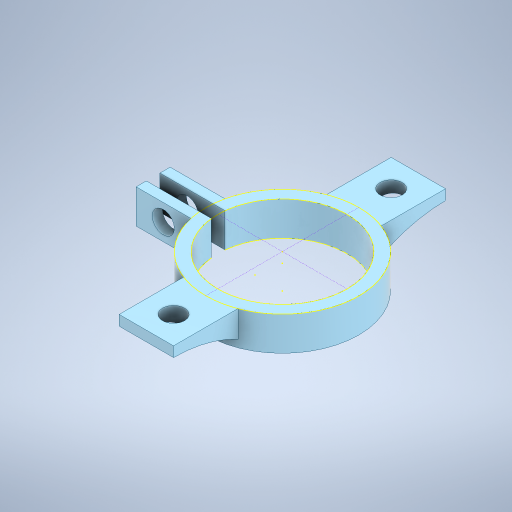
# Autodesk Inventor part: motor holder
Saved by Autodesk Inventor 2023 (Build 270158000, 158)
## iProperties
Created: 2023-04-19
Part Number: motor holder
Material: ABS Plastic
Document SubType Name: Modeling
Designer: deepa
Density: 1.06 g/cm^3
Appearance: Smooth - White
Author: deepa
Autodesk Inventor part; units mm, degrees
ref_plane "YZ Plane" through (0, 0, 0) normal (1, 0, 0) x (0, 1, 0)
ref_plane "XZ Plane" through (0, 0, 0) normal (0, 1, 0) x (-1, 0, 0)
ref_plane "XY Plane" through (0, 0, 0) normal (0, 0, 1) x (1, 0, 0)
sketch "Sketch1" plane through (0, 0, 0) normal (0, 1, 0) x (-1, 0, 0)
  circle A0 centre (0, 0) radius 22.5
  circle A1 centre (0, 0) radius 19
  dimension "d0" = 45
  dimension "d1" = 38
  constraints: 2 centre point, 1 coincident
  measures "d0" diameter of A0
  measures "d1" diameter of A1
extrude "Extrusion1" add sketch "Sketch1" along normal blind 10
sketch "Sketch2" plane through (0, 10, 0) normal (0, 1, 0) x (1, 0, 0)
  circle A0 centre (0, 0) radius 22.5 projected
  line L0 (0, -22.5) -> (0, 22.5) construction
  circle A1 centre (0, 0) radius 19 projected
  line L1 (-19, 0) -> (19, 0) construction
  constraints: 4 end point, 4 point on circle, 1 horizontal, 1 vertical
sketch "Sketch3" plane through (0, 10, 0) normal (0, 1, 0) x (1, 0, 0)
  line L0 (-8, -20) -> (8, -20)
  line L1 (8, -20) -> (8, -40)
  line L2 (8, -40) -> (-8, -40)
  line L3 (-8, -40) -> (-8, -20)
  point P0 (0, 0)
  dimension "d4" = 16
  dimension "d5" = 20
  dimension "d6" = 20
  dimension "d7" = 8
  constraints: 8 end point, 2 parallel, 1 horizontal, 1 perpendicular
  measures "d4" distance of L1.end L2.end
  measures "d5" distance from line of L0 point (0, 0)
  measures "d6" distance of L2.end L0.start
  measures "d7" distance from line of L3 point (0, 0)
extrude "Extrusion2" add sketch "Sketch3" against normal blind 3
pattern_circular "Circular Pattern1" count 2 over 360 about axis through (0, 0, 0) along (0, 1, 0) of "Extrusion2"
sketch "Sketch4" plane through (0, 10, 0) normal (0, 1, 0) x (1, 0, 0)
  point P0 (0, 0)
sketch "Sketch6" plane through (0, 10, 0) normal (0, 1, 0) x (1, 0, 0)
  line L0 (-20, 5) -> (-38, 5)
  line L1 (-38, 5) -> (-38, 2)
  line L2 (-38, 2) -> (-20, 2)
  line L3 (-20, 2) -> (-20, 5)
  point P0 (0, 0)
  dimension "d14" = 18
  dimension "d15" = 3
  dimension "d16" = 20
  dimension "d17" = 2
  constraints: 8 end point, 2 parallel, 1 horizontal, 1 perpendicular
  measures "d14" distance of L2.end L1.end
  measures "d15" distance of L1.end L0.end
  measures "d16" distance from line of L3 point (0, 0)
  measures "d17" distance from line of L2 point (0, 0)
extrude "Extrusion3" add sketch "Sketch6" against normal blind 10
pattern_linear "Rectangular Pattern1" count 2 spacing 7 along (0, 0, 1) of "Extrusion3"
sketch "Sketch7" plane through (-38, 10, 2) normal (-1, 0, 0) x (0, 0, 1)
  line L0 (0, 0) -> (0, -10) projected
  line L1 (-4, 0) -> (-4, -10) projected
  line L2 (0, -10) -> (-4, -10)
  line L3 (-4, -10) -> (-4, 0)
  line L4 (-4, 0) -> (0, 0)
  line L5 (0, 0) -> (0, -10)
  point P0 (-2, -10)
  constraints: 8 end point, 2 parallel, 1 horizontal, 1 perpendicular
extrude "Extrusion4" cut sketch "Sketch7" against normal blind 20
sketch "Sketch9" plane through (0, 7, 0) normal (0, -1, 0) x (1, 0, 0)
  point P0 (0, 0)
sketch "Sketch10" plane through (0, 7, 0) normal (0, -1, 0) x (1, 0, 0)
  point P0 (0, 0)
sketch "Sketch11" plane through (8, 10, -40) normal (0, 0, -1) x (-1, 0, 0)
  point P0 (8, -10)
sketch "Sketch13" plane through (-8, 10, -40) normal (-1, 0, 0) x (0, 0, 1)
  point P0 (40, -10)
sketch "Sketch14" plane through (-38, 10, 5) normal (0, 0, 1) x (1, 0, 0)
  circle A0 centre (8, -5) radius 3.25
  line L0 (0, 0) -> (0, -10) projected
  line L1 (16.0626, -10) -> (0, -10) projected
  point P0 (38, -10)
  dimension "d27" = 6.5
  dimension "d28" = 8
  dimension "d29" = 5
  constraints: 1 centre point
  measures "d27" diameter of A0
  measures "d28" distance from line of L0 A0.centre
  measures "d29" distance from line of L1 A0.centre
extrude "Extrusion5" cut sketch "Sketch14" against normal blind 20
sketch "Sketch17" plane through (0, 0, 0) normal (0, -1, 0) x (1, 0, 0)
  arc A0 (-21.9374, -5) -> (-8, -21.0297) centre (0, 0) ccw projected
  line L0 (-8, -21.0297) -> (-8, -17.2337) construction
  arc A1 (-18.8944, -2) -> (-18.8944, 2) centre (0, 0) ccw projected
  constraints: 2 end point, 1 point on circle, 1 vertical
sketch "Sketch21" plane through (-8, 10, -40) normal (-1, 0, 0) x (0, 0, 1)
  line L0 (0, -43) -> (18, -10) construction
  line L1 (62.5, -10) -> (17.5, -10) projected
  line L2 (18.9703, -3) -> (0, -3) projected
  line L3 (0, 0) -> (0, -3) projected
  circle A0 centre (0, -43) radius 40
  line L4 (18.9703, -3) -> (18.9703, -10)
  point P0 (40, -10)
  point P1 (45, -10)
  point P2 (35, -10)
  point P3 (18.9703, -7.7845)
  dimension "d33" = 40
  dimension "d34" = 0
  dimension "d35" = 18
  constraints: 4 end point, 2 point on line, 1 centre point, 1 coincident, 1 perpendicular, 1 tangent
  measures "d33" distance from line of L2 L0.start
  measures "d34" distance from line of L3 L0.start
  measures "d35" horizontal distance of L0.start L0.end
extrude "Extrusion6" add sketch "Sketch21" against normal blind 16 contours A0 L2 L4
sketch "Sketch22" plane through (0, 10, 0) normal (0, 1, 0) x (1, 0, 0)
  circle A0 centre (0, 32) radius 3.25
  line L0 (8, 40) -> (-8, 40) projected
  point P0 (0, 0)
  dimension "d38" = 6.5
  dimension "d39" = 8
  constraints: 1 centre point
  measures "d38" diameter of A0
  measures "d39" distance from line of L0 A0.centre
extrude "Extrusion7" cut sketch "Sketch22" against normal blind 16
pattern_circular "Circular Pattern2" count 2 over 360 about axis through (0, 0, 0) along (0, 1, 0) of "Extrusion7", "Extrusion6"
body "Solid1"
